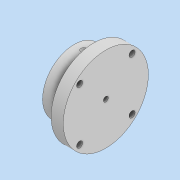
# Autodesk Inventor part: 메인 바퀴 간격링
Saved by Autodesk Inventor 2020 (Build 240168000, 168)
## iProperties
Created: 2020-05-04
Part Number: 메인 바퀴 간격링
Material: 일반
Document SubType Name: Modeling
Designer: sbahn
Density: 1 g/cm^3
Appearance: 기본값
Author: sbahn
Autodesk Inventor part; units mm, degrees
ref_plane "YZ Plane" through (0, 0, 0) normal (1, 0, 0) x (0, 1, 0)
ref_plane "XY Plane" through (0, 0, 0) normal (0, 0, 1) x (1, 0, 0)
sketch "스케치1" plane through (0, 0, 0) normal (1, 0, 0) x (0, 1, 0)
  circle A0 centre (0, 0) radius 13
  circle A1 centre (0, 0) radius 5
  dimension "d0" = 26
  dimension "d1" = 10
  constraints: 2 centre point, 2 coincident
  measures "d0" diameter of A0
  measures "d1" diameter of A1
extrude "돌출1" add sketch "스케치1" along normal blind 8
ref_plane "작업 평면1" through (0, 13, 0) normal (0, 1, 0) x (-1, 0, 0)
sketch "스케치2" plane through (0, 13, 0) normal (0, 1, 0) x (-1, 0, 0)
  line L0 (0, 0) -> (-4, 0)
  circle A0 centre (-4, 0) radius 1.25
  dimension "d4" = 4
  dimension "d5" = 2.5
  constraints: 2 coincident, 2 end point, 1 centre point, 1 horizontal
  measures "d4" distance of L0.start L0.end
  measures "d5" diameter of A0
extrude "돌출2" cut sketch "스케치2" against normal blind 8
sketch "스케치3" plane through (8, 0, 0) normal (1, 0, 0) x (0, 0, -1)
  circle A0 centre (0, 0) radius 17.5
  dimension "d8" = 35
  constraints: 1 centre point, 1 coincident
  measures "d8" diameter of A0
extrude "돌출3" add sketch "스케치3" along normal blind 5
sketch "스케치4" plane through (8, 0, 0) normal (-1, 0, 0) x (0, 0, 1)
  circle A0 centre (0, 0) radius 1
  dimension "d11" = 2
  constraints: 1 centre point, 1 coincident
  measures "d11" diameter of A0
extrude "돌출4" cut sketch "스케치4" against normal blind 5
sketch "스케치5" plane through (8, 0, 0) normal (-1, 0, 0) x (0, 0, 1)
  circle A0 centre (0, 0) radius 17.5 projected
  circle A1 centre (0, 0) radius 13 projected
  line L0 (0, 0) -> (17.5, 0)
  line L1 (0, 0) -> (12.3744, 12.3744)
  circle A2 centre (0, 0) radius 15.25
  circle A3 centre (10.7834, 10.7834) radius 1.25
  dimension "d15" = 30.5
  dimension "d14" = 45
  dimension "d16" = 2.5
  constraints: 4 end point, 2 coincident, 2 point on circle, 1 centre point, 1 horizontal, 1 point on line, 3 other
  measures "d14" angle of L0 L1
  measures "d16" diameter of A3
hole "구멍1" at (8, 10.7834, 10.7834) direction (1, 0, 0) diameter 2.5 depth 10 tip angle 118 countersink diameter 4 countersink angle 90
pattern_circular "원형 패턴1" count 4 over 360 about axis through (8, 0, 0) along (1, 0, 0) of "구멍1"
